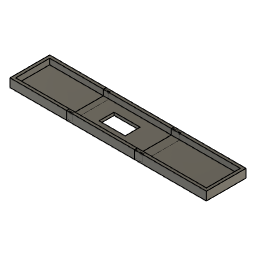
JuFo_CO2_Matrix_Kappe_v1_v6 (Autodesk Fusion 360 design; units mm, degrees)
Autodesk Fusion 360 part; units mm, degrees
sketch "Skizze1" plane through (0, 0, 0) normal (0, 0, 1) x (1, 0, 0)
  line L0 (0, 0) -> (347, 0)
  line L1 (347, 0) -> (347, 70)
  line L2 (347, 70) -> (0, 70)
  line L3 (0, 70) -> (0, 0)
  dimension "d1" = 347
  dimension "d2" = 70
  constraint horizontal L0
  constraint vertical L1
  constraint horizontal L2
  constraint vertical L3
  constraint coincident L0.start L3.end
  measures "d1" distance of L0.start L0.end
  measures "d2" distance of L0.end L1.end
extrude "Extrusion1" add sketch "Skizze1" along normal blind 15 makes body 1
shell "Schale1" thickness 5 removed faces 1 at (115.6667, 46.6667, 15) on bodies 1
sketch "Skizze2" plane through (0, 0, 5) normal (0, 0, 1) x (-1, 0, 0)
  line L0 (-5, -65) -> (-5, -5)
  line L1 (-5, -5) -> (-342, -5)
  line L2 (-342, -5) -> (-342, -65)
  line L3 (-342, -65) -> (-5, -65)
  line L4 (-134.5202, -49.3996) -> (-180.5202, -49.3996)
  line L5 (-180.5202, -49.3996) -> (-180.5202, -22.8996)
  line L6 (-180.5202, -22.8996) -> (-134.5202, -22.8996)
  line L7 (-134.5202, -22.8996) -> (-134.5202, -49.3996)
  dimension "d6" = 46
  dimension "d7" = 26.5
  constraint horizontal L4
  constraint vertical L5
  constraint horizontal L6
  constraint vertical L7
  measures "d6" distance of L4.start L4.end
  measures "d7" distance of L4 L6
extrude "Extrusion2" cut sketch "Skizze2" against normal blind 20 contours L4 L5 L6 L7 bodies 1
ref_plane "Arbeitsebene1" through (100, 0, 0) normal (1, 0, 0) x (0, 1, 0)
ref_plane "Arbeitsebene2" through (220, 0, 0) normal (1, 0, 0) x (0, 1, 0)
split "Teilen1" by plane through (100, 0, 0) normal (1, 0, 0) bodies 1 makes body 2 at (291.5067, 30.9665, 0)
split "Teilen2" by plane through (220, 0, 0) normal (1, 0, 0) bodies 2 makes body 3 at (262.3333, 46.6667, 0)
sketch "Skizze3" plane through (100, 0, 0) normal (1, 0, 0) x (0, 1, 0)
  line L0 (0, 15) -> (0, 0)
  line L1 (0, 0) -> (70, 0)
  line L2 (70, 0) -> (70, 15)
  line L3 (70, 15) -> (65, 15)
  line L4 (65, 15) -> (65, 5)
  line L5 (65, 5) -> (5, 5)
  line L6 (5, 5) -> (5, 15)
  line L7 (5, 15) -> (0, 15)
  line L8 (1.5, 1.5) -> (68.5, 1.5)
  line L9 (68.5, 1.5) -> (68.5, 13.5)
  line L10 (68.5, 13.5) -> (66.5, 13.5)
  line L11 (66.5, 13.5) -> (66.5, 3.5)
  line L12 (66.5, 3.5) -> (3.5, 3.5)
  line L13 (3.5, 3.5) -> (3.5, 13.5)
  line L14 (3.5, 13.5) -> (1.5, 13.5)
  line L15 (1.5, 13.5) -> (1.5, 1.5)
  dimension "d12" = -1.5
extrude "Extrusion3" add sketch "Skizze3" along normal blind 10 contours L8 L9 L10 L11 L12 L13 L14 L15 bodies 1
fillet "Abrundung1" radius 0.6 14 edges at (105, 1.5, 13.5) (105, 3.5, 13.5) (110, 2.5, 13.5) (110, 1.5, 7.5) (105, 1.5, 1.5) (110, 3.5, 8.5) (110, 35, 3.5) (110, 35, 1.5) (110, 66.5, 8.5) (110, 67.5, 13.5) (105, 66.5, 13.5) (105, 68.5, 13.5) (110, 68.5, 7.5) (105, 68.5, 1.5) on bodies 1
combine "Kombinieren1" operation cut target body 2 tool bodies 1 keep tools
move_face "Flächen versetzen1" offset -0.3 29 faces at (106.2667, 66.8251, 13.4333) (103.1333, 67.6333, 13.5) (103.1333, 68.2, 13.4196) (109.7275, 67.9783, 13.3966) (109.6749, 67.6333, 13.4333) (109.8966, 66.7725, 12.9783) (109.9333, 68.1749, 5.7) (110, 24.3, 2.3667) (109.9756, 66.9307, 6.3458) (109.8554, 24.4596, 3.2906) (106.2667, 68.5, 9.3) (103.1333, 66.5, 9.7667) (106.2667, 45.5, 3.5) (103.1333, 68.1749, 1.5667) (103.1333, 24.0333, 1.5) (109.7275, 67.9783, 1.6034) (109.4392, 45.9667, 1.5013) (106.2667, 3.5, 6.6333) (103.1333, 3.4993, 12.9285) (103.1333, 2.6333, 13.5) (106.2667, 1.5027, 12.957) (103.1333, 1.5, 9.3) (109.6749, 1.5667, 5.7) (109.4783, 1.6034, 13.2275) (109.7, 2.6333, 13.4196) (109.4783, 3.2275, 13.3966) (109.9756, 3.0693, 6.3458) (109.7275, 1.6034, 2.0217) (103.1333, 2.043, 1.5027) on bodies 2
sketch "Skizze4" plane through (220, 0, 0) normal (1, 0, 0) x (0, 1, 0)
  line L0 (0, 15) -> (0, 0)
  line L1 (0, 0) -> (70, 0)
  line L2 (70, 0) -> (70, 15)
  line L3 (70, 15) -> (65, 15)
  line L4 (65, 15) -> (65, 5)
  line L5 (65, 5) -> (5, 5)
  line L6 (5, 5) -> (5, 15)
  line L7 (5, 15) -> (0, 15)
  line L8 (3.5, 13.5) -> (1.5, 13.5)
  line L9 (1.5, 13.5) -> (1.5, 1.5)
  line L10 (1.5, 1.5) -> (68.5, 1.5)
  line L11 (68.5, 1.5) -> (68.5, 13.5)
  line L12 (68.5, 13.5) -> (66.5, 13.5)
  line L13 (66.5, 13.5) -> (66.5, 3.5)
  line L14 (66.5, 3.5) -> (3.5, 3.5)
  line L15 (3.5, 3.5) -> (3.5, 13.5)
  dimension "d18" = -1.5
extrude "Extrusion4" add sketch "Skizze4" along normal blind 15 contours L8 L9 L10 L11 L12 L13 L14 L15 bodies 2
fillet "Abrundung2" radius 0.6 14 edges at (227.5, 1.5, 13.5) (227.5, 3.5, 13.5) (235, 2.5, 13.5) (235, 1.5, 7.5) (235, 3.5, 8.5) (235, 35, 1.5) (235, 35, 3.5) (227.5, 1.5, 1.5) (235, 66.5, 8.5) (235, 68.5, 7.5) (235, 67.5, 13.5) (227.5, 66.5, 13.5) (227.5, 68.5, 1.5) (227.5, 68.5, 13.5) on bodies 2
combine "Kombinieren2" operation cut target body 3 tool bodies 2 keep tools
move_face "Flächen versetzen2" offset -0.3 29 faces at (224.8, 66.5, 9.7667) (224.8, 66.8251, 13.4333) (224.8, 67.6333, 13.5) (224.8, 68.2, 13.4196) (234.8966, 68.2275, 12.9783) (234.4285, 67.6333, 13.4993) (234.7275, 66.6034, 12.9783) (234.9975, 67.0452, 9.5929) (235, 24.3, 2.3667) (234.748, 68.3887, 9.3) (224.8, 68.5, 5.7) (224.8, 45.5, 3.5) (234.5384, 45.5, 3.4838) (234.7275, 67.9783, 1.6034) (224.8, 68.1749, 1.5667) (224.8, 24.0333, 1.5) (234.5553, 45.9667, 1.5204) (234.9975, 2.9548, 9.5929) (224.8, 2.0715, 1.5007) (229.6, 1.5, 9.3) (234.8966, 1.7725, 2.0217) (234.457, 1.5027, 9.3) (229.6, 3.4973, 12.957) (224.8, 2.6333, 13.5) (224.8, 1.5007, 12.9285) (234.4783, 1.6034, 13.2275) (234.457, 2.6333, 13.4973) (234.4783, 3.2275, 13.3966) (224.8, 3.5, 6.6333) on bodies 3
